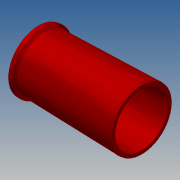
# Autodesk Inventor part: A1-19027-200-04 HCWi reducer
Saved by Autodesk Inventor 2017.3 (Build 213257000, 257)
## iProperties
Created: 2019-06-26
Part Number: A1-19027-200-04 HCWi reducer
Material: Iron, HCWI
Document SubType Name: Modeling
Designer: Graeme_Van_Dongen
Density: 7.33517 g/cm^3
Appearance: Iron Gray(1)
Mass: 1.31633e+06 g
Surface Area: 69970.9 cm^2
Volume: 179455 cm^3
Description: 28 1/2" ID x 26" ID x 2 1/16" WALL x 55 7/8" HCWI REDUCER, ASTM A532 CLASS III TYPE A, PF# 470279
Author: Graeme_Van_Dongen
Autodesk Inventor part; units mm, degrees
ref_plane "YZ Plane" through (0, 0, 0) normal (1, 0, 0) x (0, 1, 0)
ref_plane "XZ Plane" through (0, 0, 0) normal (0, 1, 0) x (-1, 0, 0)
ref_plane "XY Plane" through (0, 0, 0) normal (0, 0, 1) x (1, 0, 0)
sketch "Sketch1" plane through (0, 0, 0) normal (0, 0, 1) x (1, 0, 0)
  line L0 (0, 0) -> (1419, 0)
  line L1 (0, 330.2) -> (174.4, 330.2)
  arc A0 (174.4, 330.2) -> (182.3871, 330.3047) centre (174.4, 635) ccw
  line L2 (182.3871, 330.3047) -> (1385.6129, 361.8453)
  arc A1 (1393.6, 361.95) -> (1385.6129, 361.8453) centre (1393.6, 57.15) ccw
  line L3 (1393.6, 361.95) -> (1419, 361.95)
  line L4 (1419, 361.95) -> (1419, 412.496)
  line L5 (1419, 412.496) -> (1393.6, 412.496)
  line L6 (1393.6, 412.496) -> (1393.6, 415.925)
  line L7 (1365.025, 412.75) -> (1317.4, 412.75)
  arc A2 (1317.4, 412.75) -> (1309.4129, 412.6453) centre (1317.4, 107.95) ccw
  line L8 (1309.4129, 412.6453) -> (106.1871, 381.1047)
  arc A3 (98.2, 381) -> (106.1871, 381.1047) centre (98.2, 685.8) ccw
  line L9 (98.2, 381) -> (85.725, 381)
  line L10 (25.4, 415.925) -> (25.4, 412.496)
  line L11 (25.4, 412.496) -> (0, 412.496)
  line L12 (0, 412.496) -> (0, 330.2)
  line L13 (85.725, 381) -> (50.8, 415.925)
  line L14 (50.8, 415.925) -> (25.4, 415.925)
  line L15 (1365.025, 412.75) -> (1368.2, 415.925)
  line L16 (1368.2, 415.925) -> (1393.6, 415.925)
  dimension "d0" = 1419
  dimension "d1" = 660.4
  dimension "d2" = 723.9
  dimension "d3" = 824.992
  dimension "d4" = 50.8
  dimension "d5" = 25.4
  dimension "d6" = 25.4
  dimension "d7" = 824.992
  dimension "d8" = 762
  dimension "d9" = 25.4
  dimension "d10" = 101.6
  dimension "d11" = 304.8
  dimension "d12" = 304.8
  dimension "d13" = 1219.2
  dimension "d14" = 52.7793
  dimension "d17" = 25.4
  dimension "d18" = 45
  dimension "d19" = 831.85
  dimension "d23" = 25.4
  dimension "d24" = 45
  dimension "d25" = 831.85
  constraints: 34 end point, 8 point on circle, 8 tangent, 7 perpendicular, 4 centre point, 4 horizontal, 3 parallel, 2 equal radius, 2 point on line
  measures "d0" distance of L0.start L0.end
  measures "d1" diameter of L1 L0
  measures "d2" diameter of L3 L0
  measures "d3" diameter of L5 L0
  measures "d4" distance between parallel lines of L7 L3
  measures "d5" distance of L4.end L5.end
  measures "d6" distance of L3.start L3.end
  measures "d7" diameter of L11 L0
  measures "d8" diameter of L9 L0
  measures "d9" distance of L10.end L11.end
  measures "d10" distance from line of L4 L7.end
  measures "d11" radius of A0
  measures "d12" radius of A2
  measures "d13" horizontal distance of L3.start L1.end
  measures "d14" distance between parallel lines of L2 L8
  measures "d17" distance of L13.end L10.start
  measures "d18" angle of L14 L13
  measures "d19" diameter of L14 L0
  measures "d23" distance of L15.end L6.end
  measures "d24" angle of L16 L15
  measures "d25" diameter of L16 L0
revolve "Revolution1" add sketch "Sketch1" angle 360 about axis through (0, 0, 0) along (1, 0, 0)
fillet "Fillet1" radius 0.7937 2 edges at (1393.6, -412.496, 0) (25.4, -412.496, 0)
body "Solid1"
